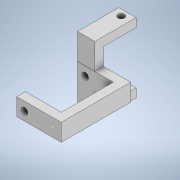
# Autodesk Inventor part: Part1_New
Saved by Autodesk Inventor 2022 (Build 260153000, 153)
## iProperties
Created: 2021-06-22
Part Number: Part1_New
Material: Generic
Document SubType Name: Modeling
Designer: athar
Density: 1 g/cm^3
Appearance: Default
Author: athar
Autodesk Inventor part; units mm, degrees
ref_plane "YZ Plane" through (0, 0, 0) normal (1, 0, 0) x (0, 1, 0)
ref_plane "XZ Plane" through (0, 0, 0) normal (0, 1, 0) x (-1, 0, 0)
ref_plane "XY Plane" through (0, 0, 0) normal (0, 0, 1) x (1, 0, 0)
sketch "Sketch1" plane through (0, 0, 0) normal (1, 0, 0) x (0, 1, 0)
  line L0 (9.8314, 40.3372) -> (-10.4886, 40.3372)
  line L1 (-10.4886, 40.3372) -> (-10.4886, -40.9428)
  line L2 (-10.4886, -40.9428) -> (9.8314, -40.9428)
  line L3 (9.8314, -40.9428) -> (9.8314, 40.3372)
  point P0 (0, 0)
  dimension "d0" = 20.32
  dimension "d1" = 81.28
  constraints: 8 end point, 2 parallel, 1 horizontal, 1 perpendicular
  measures "d0" distance of L2.end L1.end
  measures "d1" distance of L1.end L0.end
extrude "Extrusion1" add sketch "Sketch1" along normal blind 10.16
sketch "Sketch2" plane through (0, -10.4886, 40.3372) normal (0, 0, 1) x (1, 0, 0)
  point P0 (0, 10.4886)
sketch "Sketch3" plane through (0, -10.4886, 40.3372) normal (0, 0, 1) x (1, 0, 0)
  line L0 (10.16, 0) -> (10.16, 20.32) projected
  line L1 (10.16, 20.32) -> (-41.91, 20.32)
  line L2 (-41.91, 20.32) -> (-41.91, 0)
  line L3 (-41.91, 0) -> (10.16, 0)
  line L4 (10.16, 0) -> (10.16, 20.32)
  point P0 (0, 10.4886)
  dimension "d4" = 52.07
  constraints: 8 end point, 2 parallel, 1 horizontal, 1 perpendicular
  measures "d4" distance of L3.end L2.end
extrude "Extrusion2" add sketch "Sketch3" against normal blind 10.16
sketch "Sketch4" plane through (0, -10.4886, -40.9428) normal (0, 0, -1) x (-1, 0, 0)
  line L0 (41.91, 20.32) -> (-10.16, 20.32) projected
  line L1 (41.91, 0) -> (-10.16, 0) projected
  line L2 (-10.16, 20.32) -> (21.59, 20.32)
  line L3 (21.59, 20.32) -> (21.59, 0)
  line L4 (21.59, 0) -> (-10.16, 0)
  line L5 (-10.16, 0) -> (-10.16, 20.32)
  point P0 (0, 10.4886)
  dimension "d7" = 31.75
  constraints: 8 end point, 2 parallel, 1 horizontal, 1 perpendicular, 1 point on line
  measures "d7" distance of L3.end L4.end
extrude "Extrusion3" add sketch "Sketch4" against normal blind 10.16
sketch "Sketch5" plane through (10.16, -10.4886, -40.9428) normal (0, 0, -1) x (-1, 0, 0)
  point P0 (10.16, 10.4886)
sketch "Sketch6" plane through (10.16, -10.4886, -40.9428) normal (0, 0, -1) x (-1, 0, 0)
  line L0 (52.07, 20.32) -> (10.16, 20.32) projected
  line L1 (31.7479, 20.32) -> (52.0679, 20.32)
  line L2 (52.0679, 20.32) -> (52.0679, 0)
  line L3 (52.0679, 0) -> (31.7479, 0)
  line L4 (31.7479, 0) -> (31.7479, 20.32)
  point P0 (10.16, 10.4886)
  dimension "d10" = 20.32
  dimension "d11" = 20.32
  constraints: 8 end point, 2 parallel, 1 horizontal, 1 perpendicular, 1 point on line
  measures "d10" distance of L2.end L3.end
  measures "d11" distance of L1.end L2.end
sketch "Sketch7" plane through (10.16, -10.4886, -40.9428) normal (0, 0, -1) x (-1, 0, 0)
  line L0 (31.7541, 50.8916) -> (52.0741, 50.8916)
  line L1 (52.0741, 50.8916) -> (52.0741, 20.4116)
  line L2 (52.0741, 20.4116) -> (31.7541, 20.4116)
  line L3 (31.7541, 20.4116) -> (31.7541, 50.8916)
  point P0 (10.16, 10.4886)
  dimension "d12" = 20.32
  dimension "d13" = 30.48
  constraints: 8 end point, 2 parallel, 1 horizontal, 1 perpendicular
  measures "d12" distance of L1.end L2.end
  measures "d13" distance of L0.end L1.end
sketch "Sketch8" plane through (10.16, -10.4886, -40.9428) normal (0, 0, -1) x (-1, 0, 0)
  line L0 (10.16, 0) -> (52.07, 0) projected
  line L1 (31.7509, 0) -> (52.0709, 0)
  line L2 (52.0709, 0) -> (52.0709, -30.48)
  line L3 (52.0709, -30.48) -> (31.7509, -30.48)
  line L4 (31.7509, -30.48) -> (31.7509, 0)
  point P0 (10.16, 10.4886)
  dimension "d14" = 20.32
  dimension "d15" = 30.48
  constraints: 8 end point, 2 parallel, 1 horizontal, 1 perpendicular, 1 point on line
  measures "d14" distance of L2.end L3.end
  measures "d15" distance of L1.end L2.end
extrude "Extrusion4" add sketch "Sketch7" against normal blind 10.16
extrude "Extrusion5" add sketch "Sketch8" against normal blind 10.16
extrude "Extrusion6" add sketch "Sketch6" against normal blind 10.16
sketch "Sketch9" plane through (10.16, -10.4886, -40.9428) normal (0, 0, -1) x (-1, 0, 0)
  line L0 (31.7541, 20.4116) -> (31.7541, 50.8916) projected
  line L1 (31.7541, 50.8916) -> (52.0741, 50.8916)
  line L2 (52.0741, 50.8916) -> (52.0741, 40.7316)
  line L3 (52.0741, 40.7316) -> (31.7541, 40.7316)
  line L4 (31.7541, 40.7316) -> (31.7541, 50.8916)
  line L5 (31.7509, -30.48) -> (31.7509, 0) projected
  line L6 (31.7509, -30.48) -> (52.0709, -30.48)
  line L7 (52.0709, -30.48) -> (52.0709, -20.32)
  line L8 (52.0709, -20.32) -> (31.7509, -20.32)
  line L9 (31.7509, -20.32) -> (31.7509, -30.48)
  point P0 (10.16, 10.4886)
  dimension "d22" = 20.32
  dimension "d23" = 10.16
  dimension "d24" = 20.32
  dimension "d25" = 10.16
  constraints: 16 end point, 4 parallel, 2 horizontal, 2 perpendicular
  measures "d22" distance of L2.end L3.end
  measures "d23" distance of L1.end L2.end
  measures "d24" distance of L8.end L7.end
  measures "d25" distance of L7.end L6.end
extrude "Extrusion7" add sketch "Sketch9" along normal blind 38.1
sketch "Sketch10" plane through (-41.9141, 40.4029, -30.7828) normal (0, 1, 0) x (1, 0, 0)
  line L0 (0.0032, 48.26) -> (20.3232, 48.26) projected
  circle A0 centre (10.1632, 40.9995) radius 3.81
  point P0 (41.9141, -30.7828)
  point P1 (10.1632, 48.26)
  dimension "d28" = 7.62
  constraints: 1 centre point, 1 coincident, 1 midpoint
  measures "d28" diameter of A0
hole "Hole1" at (-31.7509, 40.4029, -71.7822) direction (0, -1, 0) diameter 7.62 depth 89.3191 tip angle 118
sketch "Sketch11" plane through (10.16, -10.4886, 40.3372) normal (0, 0, 1) x (1, 0, 0)
  circle A0 centre (-42.9384, 10.16) radius 3.81
  point P0 (-10.16, 10.4886)
  dimension "d36" = 7.62
  constraints: 1 centre point, 1 coincident
  measures "d36" diameter of A0
hole "Hole2" at (-32.7784, -0.3286, 40.3372) direction (0, 0, -1) diameter 7.62 depth 89.3191 tip angle 118
equation "\"d29\" = d28"
equation "\"d37\" = d28"
body "Solid1"
